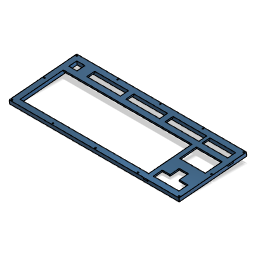
k5 top v3 (Autodesk Fusion 360 design; units mm, degrees)
Autodesk Fusion 360 part; units mm, degrees
sketch "Sketch1" plane through (0, 0, 0) normal (0, 1, 0) x (1, 0, 0)
  line L0 (0, 0) -> (371.813, 0)
  line L1 (371.813, 0) -> (371.813, 148.426)
  line L2 (371.813, 148.426) -> (0, 148.426)
  line L3 (0, 148.426) -> (0, 0)
  dimension "d1" = 371.813
  dimension "d2" = 148.426
  constraint horizontal L0
  constraint vertical L1
  constraint horizontal L2
  constraint vertical L3
  constraint coincident L0.start L3.end
  measures "d1" distance of L0.start L0.end
  measures "d2" distance of L0.start L2.end
extrude "Extrude1" add sketch "Sketch1" along normal blind 8
sketch "Sketch2" plane through (0, 8, 0) normal (0, 1, 0) x (-1, 0, 0)
  line L0 (0, -148.426) -> (0, 0)
  line L1 (0, 0) -> (-371.813, 0)
  line L2 (-371.813, 0) -> (-371.813, -148.426)
  line L3 (-371.813, -148.426) -> (0, -148.426)
  line L4 (-12, -12) -> (-359.813, -12)
  line L5 (-359.813, -12) -> (-359.813, -136.426)
  line L6 (-359.813, -136.426) -> (-12, -136.426)
  line L7 (-12, -136.426) -> (-12, -12)
  dimension "d5" = -12
extrude "Extrude2" cut sketch "Sketch2" against normal blind 50 contours L4 L5 L6 L7
fillet "Fillet1" radius 0.3 1 edges at (371.813, 4, 0)
fillet "Fillet2" radius 0.3 3 edges at (0, 4, 0) (371.813, 4, -148.426) (0, 4, -148.426)
move_body "Move1" bodies 1 to x (1, 0, 0) y (0, 1, 0) z (0, 0, 1) at (184.4687, 111.7703, -377.3274)
move_body "Move2" bodies 1 to x (1, 0, 0) y (0, 0.996195, 0.087156) z (0, -0.087156, 0.996195) at (-195.7576, -129.0647, 379.5394)
move_body "Move3" bodies 1 to x (1, 0, 0) y (0, 1, 0) z (0, 0, 1) at (-0.9057, -0.2814, -0.0438)
move_body "Move4" bodies 1 to x (1, 0, 0) y (0, 0.996195, -0.087156) z (0, 0.087156, 0.996195) at (0, 11.7731, 2.609)
move_body "Move5" bodies 1 to x (1, 0, 0) y (0, 1, 0) z (0, 0, 1) at (0, -27, 0)
sketch "Sketch3" plane through (0, 8.7648, 0) normal (0, 1, 0) x (-1, 0, 0)
sketch "Sketch4" plane through (0, 8.7648, 0) normal (0, 1, 0) x (-1, 0, 0)
sketch "Sketch5" plane through (0, 8.7648, 0) normal (0, 1, 0) x (-1, 0, 0)
sketch "Sketch6" plane through (0, 8.7648, 0) normal (0, 1, 0) x (-1, 0, 0)
  line L0 (-2, -106) -> (-2, -104.6)
  line L1 (-2, -104.6) -> (6, -104.6)
  line L2 (-2, -91) -> (-2, -92.4)
  line L3 (-2, -92.4) -> (-1.5199, -92.4)
  line L4 (-1.5199, -92.4) -> (6, -92.4)
  line L5 (6, -104.6) -> (-359.6345, -104.6)
  line L6 (-359.6345, -104.6) -> (-359.6345, -92.4)
  line L7 (-359.6345, -92.4) -> (6, -92.4)
  line L8 (6, -92.4) -> (6, -104.6)
  line L9 (6, -104.6) -> (12.1952, -104.6)
  line L10 (12.1952, -104.6) -> (12.1952, -92.4)
  line L11 (12.1952, -92.4) -> (6, -92.4)
  line L12 (6, -92.4) -> (6, -104.6)
  line L13 (-16.1747, -112.31) -> (-17.5747, -112.31)
  line L14 (-40.451, -111.5634) -> (-39.051, -111.5634)
  line L15 (-17.5747, -112.31) -> (-17.5747, -104.6)
  line L16 (-17.5747, -104.6) -> (-39.051, -104.6)
  line L17 (-39.051, -104.6) -> (-39.051, -133.7894)
  line L18 (-39.051, -133.7894) -> (-17.5747, -133.7894)
  line L19 (-17.5747, -133.7894) -> (-17.5747, -104.6)
  line L20 (-111.4212, -112.3612) -> (-112.8212, -112.3612)
  line L21 (-126.1454, -112.3612) -> (-124.7454, -112.3612)
  line L22 (-112.8212, -112.3612) -> (-112.8212, -104.6)
  line L23 (-112.8212, -104.6) -> (-124.6352, -104.6)
  line L24 (-124.6352, -104.6) -> (-124.6352, -133.8058)
  line L25 (-124.6352, -133.8058) -> (-112.8212, -133.8058)
  line L26 (-112.8212, -133.8058) -> (-112.8212, -104.6)
  line L27 (-197.2, -112.2) -> (-198.6, -112.2)
  line L28 (-212, -113) -> (-210.6, -113)
  line L29 (-198.6, -112.2) -> (-198.6, -104.6)
  line L30 (-198.6, -104.6) -> (-210.5821, -104.6)
  line L31 (-210.5821, -104.6) -> (-210.5821, -133.6521)
  line L32 (-210.5821, -133.6521) -> (-198.6, -133.6521)
  line L33 (-198.6, -133.6521) -> (-198.6, -104.6)
  line L34 (-282.9, -111.1) -> (-284.3, -111.1)
  line L35 (-292.8, -111) -> (-291.4, -111)
  line L36 (-284.3, -111.1) -> (-284.3, -104.6)
  line L37 (-284.3, -104.6) -> (-291.412, -104.6)
  line L38 (-291.412, -104.6) -> (-291.412, -133.8732)
  line L39 (-291.412, -133.8732) -> (-284.3, -133.8732)
  line L40 (-284.3, -133.8732) -> (-284.3, -104.6)
  line L41 (-280, -82) -> (-281.4, -82)
  line L42 (-281.4, -82) -> (-281.4, -83)
  line L43 (-281.4, -83) -> (-281.4, -92.4)
  line L44 (-292.8378, -81.526) -> (-291.4378, -81.526)
  line L45 (-291.4378, -81.526) -> (-291.4378, -92.4)
  line L46 (-281.4, -92.4) -> (-291.4378, -92.4)
  line L47 (-291.4378, -92.4) -> (-291.4378, 14.6553)
  line L48 (-291.4378, 14.6553) -> (-281.4, 14.6553)
  line L49 (-281.4, 14.6553) -> (-281.4, -92.4)
  line L50 (-293.5485, -55.1894) -> (-291.4378, -55.1894)
  line L51 (-293.5485, -55.1894) -> (-359.6, -55.1894)
  line L52 (-328.5187, -17.2027) -> (-359.611, -17.2027)
  line L53 (-359.611, -17.2027) -> (-359.6, -55.1894)
  line L54 (-293.5612, -17.1732) -> (-291.4378, -17.1732)
  line L55 (-293.5612, -17.1732) -> (-308.5612, -17.1732)
  line L56 (-308.5612, -17.1732) -> (-308.5612, -37.1678)
  line L57 (-308.5612, -37.1678) -> (-328.55, -37.1678)
  line L58 (-328.55, -37.1678) -> (-328.5734, -37.1678)
  line L59 (-328.5734, -37.1678) -> (-328.5187, -17.2027)
  dimension "d13" = 1.4
  dimension "d14" = 1.4
  dimension "d15" = 12.2
  dimension "d16" = 1.4
  dimension "d17" = 1.4
  dimension "d18" = 1.4
  dimension "d19" = 1.4
  dimension "d20" = 1.4
  dimension "d21" = 1.4
  dimension "d22" = 1.4
  dimension "d23" = 1.4
  dimension "d24" = 1.4
  dimension "d25" = 1.4
  dimension "d26" = 15
  constraint vertical L0
  constraint perpendicular L0 L1
  constraint perpendicular L1 L2
  constraint perpendicular L2 L3
  constraint perpendicular L2 L4
  constraint horizontal L5
  constraint vertical L6
  constraint horizontal L7
  constraint vertical L8
  constraint horizontal L9
  constraint vertical L10
  constraint horizontal L11
  constraint vertical L12
  constraint horizontal L13
  constraint horizontal L14
  constraint coincident L5 L15.end
  constraint perpendicular L5 L15
  constraint horizontal L16
  constraint vertical L17
  constraint horizontal L18
  constraint vertical L19
  constraint horizontal L20
  constraint horizontal L21
  constraint coincident L5 L22.end
  constraint perpendicular L5 L22
  constraint horizontal L23
  constraint vertical L24
  constraint horizontal L25
  constraint vertical L26
  constraint parallel L5 L27
  constraint horizontal L28
  constraint coincident L5 L29.end
  constraint perpendicular L5 L29
  constraint horizontal L30
  constraint vertical L31
  constraint horizontal L32
  constraint vertical L33
  constraint horizontal L34
  constraint horizontal L35
  constraint coincident L5 L36.end
  constraint perpendicular L5 L36
  constraint horizontal L37
  constraint vertical L38
  constraint horizontal L39
  constraint vertical L40
  constraint parallel L7 L41
  constraint perpendicular L41 L42
  constraint coincident L7 L43.end
  constraint perpendicular L7 L43
  constraint parallel L7 L44
  constraint coincident L7 L45.end
  constraint perpendicular L7 L45
  constraint horizontal L46
  constraint vertical L47
  constraint horizontal L48
  constraint vertical L49
  constraint coincident L47 L50.end
  constraint perpendicular L47 L50
  constraint perpendicular L47 L51
  constraint horizontal L52
  constraint coincident L47 L54.end
  constraint perpendicular L47 L54
  constraint perpendicular L47 L55
  constraint perpendicular L55 L56
  constraint perpendicular L56 L57
  constraint perpendicular L56 L58
  measures "d13" distance of L0.start L0.end
  measures "d14" distance of L2.start L2.end
  measures "d15" distance of L1.end L4.end
  measures "d16" distance of L13.start L13.end
  measures "d17" distance of L14.start L14.end
  measures "d18" distance of L20.start L20.end
  measures "d19" distance of L21.start L21.end
  measures "d20" distance of L27.start L27.end
  measures "d21" distance of L28.start L28.end
  measures "d22" distance of L34.start L34.end
  measures "d23" distance of L35.start L35.end
  measures "d24" distance of L41.start L41.end
  measures "d25" distance of L44.start L44.end
  measures "d26" distance of L54.start L55.end
extrude "Extrude3" add sketch "Sketch6" against normal blind 3.2
move_body "Move6" bodies 1 to x (1, 0, 0) y (0, 0.996195, 0.087156) z (0, -0.087156, 0.996195) at (76.1693, -5.6461, -273.3125)
sketch "Sketch7" plane through (0, -41.4595, -3.6272) normal (0, -0.996195, -0.087156) x (-1, 0, 0)
  arc A0 (-435.5161, 405.6163) -> (-435.8161, 405.3163) centre (-435.5161, 405.3163) ccw
  line L0 (-435.8161, 405.3163) -> (-435.8161, 257.4678)
  arc A1 (-435.8161, 257.4678) -> (-435.5161, 257.1678) centre (-435.5161, 257.4678) ccw
  line L1 (-435.5161, 257.1678) -> (-64.3031, 257.1678)
  arc A2 (-64.3031, 257.1678) -> (-64.0031, 257.4678) centre (-64.3031, 257.4678) ccw
  line L2 (-64.0031, 257.4678) -> (-64.0031, 405.3163)
  arc A3 (-64.0031, 405.3163) -> (-64.3031, 405.6163) centre (-64.3031, 405.3163) ccw
  line L3 (-64.3031, 405.6163) -> (-435.5161, 405.6163)
  circle A4 centre (-67.0031, 402.6163) radius 1.5
  circle A5 centre (-249.9096, 402.6163) radius 1.5
  circle A6 centre (-432.8161, 402.6163) radius 1.5
  circle A7 centre (-342.9564, 260.2434) radius 1.5
  circle A8 centre (-67.0031, 260.1678) radius 1.5
  circle A9 centre (-249.9096, 260.1678) radius 1.5
  circle A10 centre (-156.671, 260.5139) radius 1.5
  circle A11 centre (-432.7611, 260.2018) radius 1.5
  circle A12 centre (-432.8493, 331.3921) radius 1.5
  circle A13 centre (-342.9564, 402.5847) radius 1.5
  circle A14 centre (-156.671, 402.6163) radius 1.5
  circle A15 centre (-66.9931, 331.3921) radius 1.5
  line L4 (-423.8161, 393.6163) -> (-76.0031, 393.6163)
  line L5 (-76.0031, 393.6163) -> (-76.0031, 269.1678)
  line L6 (-76.0031, 269.1678) -> (-423.8161, 269.1678)
  line L7 (-423.8161, 269.1678) -> (-423.8161, 393.6163)
  circle A16 centre (-432.8161, 402.6163) radius 1.5
  circle A17 centre (-342.9564, 402.5847) radius 1.5
  circle A18 centre (-249.9096, 402.6163) radius 1.5
  circle A19 centre (-156.671, 402.6163) radius 1.5
  circle A20 centre (-67.0031, 402.6163) radius 1.5
  circle A21 centre (-66.9931, 331.3921) radius 1.5
  circle A22 centre (-67.0031, 260.1678) radius 1.5
  circle A23 centre (-156.671, 260.5139) radius 1.5
  circle A24 centre (-249.9096, 260.1678) radius 1.5
  circle A25 centre (-342.9564, 260.2434) radius 1.5
  circle A26 centre (-432.7611, 260.2018) radius 1.5
  circle A27 centre (-432.8493, 331.3921) radius 1.5
  constraint concentric A6 A16
  constraint concentric A13 A17
  constraint concentric A5 A18
  constraint concentric A14 A19
  constraint concentric A4 A20
  constraint concentric A15 A21
  constraint concentric A8 A22
  constraint concentric A10 A23
  constraint concentric A9 A24
  constraint concentric A7 A25
  constraint concentric A11 A26
  constraint concentric A12 A27
hole "Hole1" at (432.7611, -18.7814, -262.8388) at (342.9564, -18.7778, -262.8803) at (249.9096, -18.7844, -262.805) at (156.671, -18.7542, -263.1498) at (67.0031, -18.7844, -262.805) at (66.9931, -12.5768, -333.7583) at (67.0031, -6.3692, -404.7115) at (156.671, -6.3692, -404.7115) at (249.9096, -6.3692, -404.7115) at (342.9564, -6.3719, -404.68) at (432.8161, -6.3692, -404.7115) at (432.8493, -12.5768, -333.7583) direction (0, 0.996195, 0.087156) diameter 3 depth 90 tip angle 118
